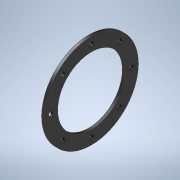
# Autodesk Inventor part: MountingRing
Saved by Autodesk Inventor 2020 (Build 240168000, 168)
## iProperties
Created: 2019-11-13
Part Number: MountingRing
Material: Generic
Document SubType Name: Modeling
Designer: nicoc
Density: 1 g/cm^3
Appearance: Glossy - Black
Author: nicoc
Autodesk Inventor part; units mm, degrees
ref_plane "YZ Plane" through (0, 0, 0) normal (1, 0, 0) x (0, 1, 0)
ref_plane "XZ Plane" through (0, 0, 0) normal (0, 1, 0) x (-1, 0, 0)
ref_plane "XY Plane" through (0, 0, 0) normal (0, 0, 1) x (1, 0, 0)
sketch "Sketch1" plane through (0, 0, 0) normal (1, 0, 0) x (0, 1, 0)
  circle A0 centre (175, -175) radius 175
  point P0 (0, 0)
  dimension "d0" = 175
  dimension "d1" = 175
  dimension "d2" = 350
  constraints: 1 centre point
  measures "d0" horizontal distance of A0.centre point (0, 0)
  measures "d1" horizontal distance of A0.centre point (0, 0)
  measures "d2" diameter of A0
extrude "Extrusion1" add sketch "Sketch1" along normal blind 10
sketch "Sketch2" plane through (10, 175, -175) normal (1, 0, 0) x (0, 0, -1)
  circle A0 centre (0, 0) radius 125
  point P0 (-175, -175)
  dimension "d5" = 250
  constraints: 1 centre point
  measures "d5" diameter of A0
extrude "Extrusion2" cut sketch "Sketch2" against normal through all
sketch "Sketch3" plane through (10, 175, -175) normal (1, 0, 0) x (0, 0, -1)
  circle A0 centre (0, 0) radius 175 projected
  point P0 (-175, -175)
  point P1 (-150, 0)
  dimension "d8" = 150
  dimension "d9" = 0
  measures "d8" distance of A0.centre point (-150, 0)
  measures "d9" vertical distance of A0.centre point (-150, 0)
hole "Hole1" at (10, 175, -25) direction (-1, 0, 0) diameter 17 end through all
pattern_circular "Circular Pattern1" count 8 over 360 about axis through (10, 175, -175) along (-1, 0, 0) of "Hole1"
sketch "Sketch5" plane through (0, 175, -175) normal (-1, 0, 0) x (0, 0, 1)
  circle A0 centre (0, 0) radius 125 construction
  line L0 (228.602, 0) -> (0, 0) construction
  line L1 (0, 0) -> (225.8114, -82.1886) construction
  arc A1 (140.9539, -51.303) -> (150, 0) centre (0, 0) ccw construction
  arc A2 (148.9413, -54.2102) -> (158.5, 0) centre (0, 0) ccw
  arc A3 (132.9665, -48.3959) -> (141.5, 0) centre (0, 0) ccw
  arc A4 (132.9665, -48.3959) -> (148.9413, -54.2102) centre (140.9539, -51.303) ccw
  arc A5 (158.5, 0) -> (141.5, 0) centre (150, 0) ccw
  circle A6 centre (0, 0) radius 125 construction
  line L2 (228.602, 0) -> (0, 0) construction
  line L3 (0, 0) -> (225.8114, -82.1886) construction
  arc A7 (140.9539, -51.303) -> (150, 0) centre (0, 0) ccw construction
  arc A8 (148.9413, -54.2102) -> (158.5, 0) centre (0, 0) ccw
  arc A9 (132.9665, -48.3959) -> (141.5, 0) centre (0, 0) ccw
  arc A10 (132.9665, -48.3959) -> (148.9413, -54.2102) centre (140.9539, -51.303) ccw
  arc A11 (158.5, 0) -> (141.5, 0) centre (150, 0) ccw
  point P0 (175, -175)
  point P1 (175, -175)
  dimension "d30" = 20
  dimension "d31" = 150
  dimension "d32" = 8.5
  dimension "d33" = 8.5
  dimension "d34" = 8.5
  dimension "d35" = 8.5
  dimension "d38" = 20
  dimension "d39" = 150
  dimension "d40" = 8.5
  dimension "d41" = 8.5
  dimension "d42" = 8.5
  dimension "d43" = 8.5
  constraints: 20 point on circle, 11 centre point, 8 end point, 6 coincident, 4 point on line, 2 horizontal
  measures "d30" angle of L0 L1
  measures "d31" radius of A1
  measures "d32" radial gap between concentric circles of A2 A1
  measures "d33" radial gap between concentric circles of A3 A1
  measures "d34" radius of A4
  measures "d35" radius of A5
  measures "d38" angle of L2 L3
  measures "d39" radius of A7
  measures "d40" radial gap between concentric circles of A8 A7
  measures "d41" radial gap between concentric circles of A9 A7
  measures "d42" radius of A10
  measures "d43" radius of A11
extrude "Extrusion3" cut sketch "Sketch5" against normal blind 5
equation "\"d33\" = d32"
equation "\"d34\" = d32"
equation "\"d35\" = d32"
equation "\"d41\" = d40"
equation "\"d42\" = d40"
equation "\"d43\" = d40"
body "Solid1"
